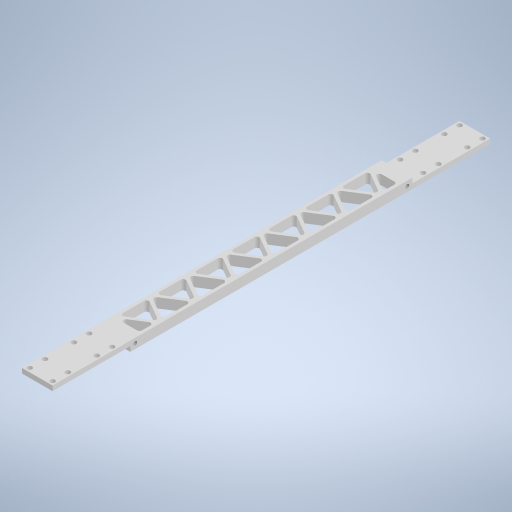
# Autodesk Inventor part: Connector Plate
Saved by Autodesk Inventor 2023 (Build 270158000, 158)
## iProperties
Created: 2022-09-25
Part Number: Connector Plate
Material: Generic
Document SubType Name: Modeling
Designer: deli
Density: 1 g/cm^3
Appearance: Default
Author: deli
Autodesk Inventor part; units mm, degrees
ref_plane "YZ Plane" through (0, 0, 0) normal (1, 0, 0) x (0, 1, 0)
ref_plane "XZ Plane" through (0, 0, 0) normal (0, 1, 0) x (-1, 0, 0)
ref_plane "XY Plane" through (0, 0, 0) normal (0, 0, 1) x (1, 0, 0)
sketch "Sketch1" plane through (0, 0, 0) normal (0, 1, 0) x (-1, 0, 0)
  line L0 (25.6456, 316.5178) -> (5.6456, 316.5178)
  line L1 (5.6456, 316.5178) -> (5.6456, 30.4178)
  line L2 (5.6456, 30.4178) -> (25.6456, 30.4178)
  line L3 (25.6456, 30.4178) -> (25.6456, 316.5178)
  circle A0 centre (23.1456, 314.0178) radius 1.6
  circle A1 centre (23.1456, 304.0178) radius 1.6
  circle A2 centre (8.1456, 314.0178) radius 1.6
  circle A3 centre (8.1456, 304.0178) radius 1.6
  line L4 (23.1456, 314.0178) -> (23.1456, 304.0178) construction
  line L5 (23.1456, 304.0178) -> (8.1456, 304.0178) construction
  line L6 (8.1456, 304.0178) -> (8.1456, 314.0178) construction
  line L7 (8.1456, 314.0178) -> (23.1456, 314.0178) construction
  circle A4 centre (23.1456, 285.1178) radius 1.6
  circle A5 centre (23.1456, 275.1178) radius 1.6
  circle A6 centre (8.1456, 285.1178) radius 1.6
  circle A7 centre (8.1456, 275.1178) radius 1.6
  line L8 (23.1456, 285.1178) -> (23.1456, 275.1178) construction
  line L9 (23.1456, 275.1178) -> (8.1456, 275.1178) construction
  line L10 (8.1456, 275.1178) -> (8.1456, 285.1178) construction
  line L11 (8.1456, 285.1178) -> (23.1456, 285.1178) construction
  circle A8 centre (23.1456, 71.8178) radius 1.6
  circle A9 centre (23.1456, 61.8178) radius 1.6
  circle A10 centre (8.1456, 71.8178) radius 1.6
  circle A11 centre (8.1456, 61.8178) radius 1.6
  line L12 (23.1456, 71.8178) -> (23.1456, 61.8178) construction
  line L13 (23.1456, 61.8178) -> (8.1456, 61.8178) construction
  line L14 (8.1456, 61.8178) -> (8.1456, 71.8178) construction
  line L15 (8.1456, 71.8178) -> (23.1456, 71.8178) construction
  circle A12 centre (23.1456, 42.9178) radius 1.6
  circle A13 centre (23.1456, 32.9178) radius 1.6
  circle A14 centre (8.1456, 42.9178) radius 1.6
  circle A15 centre (8.1456, 32.9178) radius 1.6
  line L16 (23.1456, 42.9178) -> (23.1456, 32.9178) construction
  line L17 (23.1456, 32.9178) -> (8.1456, 32.9178) construction
  line L18 (8.1456, 32.9178) -> (8.1456, 42.9178) construction
  line L19 (8.1456, 42.9178) -> (23.1456, 42.9178) construction
  line L20 (7.6456, 76.6425) -> (23.6456, 76.6425)
  line L21 (23.6456, 89.1783) -> (7.6456, 79.0121)
  line L22 (7.6456, 76.6425) -> (7.6456, 269.3043) construction
  line L23 (23.6456, 76.6425) -> (23.6456, 269.3043) construction
  line L24 (7.6456, 269.3043) -> (23.6456, 269.3043)
  line L25 (23.6456, 89.1783) -> (7.6456, 98.4159)
  line L26 (7.6456, 79.0121) -> (7.6456, 98.4159)
  line L27 (23.6456, 91.4877) -> (7.6456, 100.7253)
  line L28 (23.6456, 110.8914) -> (7.6456, 100.7253)
  line L29 (23.6456, 91.4877) -> (23.6456, 110.8914)
  line L30 (7.6456, 103.0948) -> (23.6456, 113.261)
  line L31 (23.6456, 113.261) -> (7.6456, 122.4986)
  line L32 (7.6456, 122.4986) -> (7.6456, 103.0948)
  line L33 (23.6456, 115.5704) -> (7.6456, 124.808)
  line L34 (7.6456, 124.808) -> (23.6456, 134.9741)
  line L35 (23.6456, 134.9741) -> (23.6456, 115.5704)
  line L36 (23.6456, 137.3437) -> (7.6456, 127.1775)
  line L37 (7.6456, 127.1775) -> (7.6456, 146.5813)
  line L38 (23.6456, 137.3437) -> (7.6456, 146.5813)
  line L39 (23.6456, 139.6531) -> (7.6456, 148.8907)
  line L40 (7.6456, 148.8907) -> (23.6456, 159.0568)
  line L41 (23.6456, 159.0568) -> (23.6456, 139.6531)
  line L42 (7.6456, 151.2603) -> (23.6456, 161.4264)
  line L43 (23.6456, 161.4264) -> (7.6456, 170.664)
  line L44 (7.6456, 151.2603) -> (7.6456, 170.664)
  line L45 (7.6456, 172.9734) -> (23.6456, 163.7358)
  line L46 (23.6456, 163.7358) -> (23.6456, 183.1396)
  line L47 (23.6456, 183.1396) -> (7.6456, 172.9734)
  line L48 (7.6456, 175.343) -> (23.6456, 185.5091)
  line L49 (23.6456, 185.5091) -> (7.6456, 194.7467)
  line L50 (7.6456, 175.343) -> (7.6456, 194.7467)
  line L51 (7.6456, 76.6425) -> (23.6456, 86.8087)
  line L52 (23.6456, 187.8185) -> (7.6456, 197.0561)
  line L53 (7.6456, 197.0561) -> (23.6456, 207.2223)
  line L54 (23.6456, 187.8185) -> (23.6456, 207.2223)
  line L55 (23.6456, 209.5918) -> (7.6456, 199.4257)
  line L56 (7.6456, 199.4257) -> (7.6456, 218.8294)
  line L57 (7.6456, 218.8294) -> (23.6456, 209.5918)
  line L58 (23.6456, 211.9012) -> (7.6456, 221.1388)
  line L59 (7.6456, 221.1388) -> (23.6456, 231.305)
  line L60 (23.6456, 231.305) -> (23.6456, 205.5717)
  line L61 (7.6456, 223.5084) -> (23.6456, 233.6746)
  line L62 (23.6456, 233.6746) -> (7.6456, 242.9122)
  line L63 (7.6456, 242.9122) -> (7.6456, 223.5084)
  line L64 (7.6456, 245.2216) -> (23.6456, 235.984)
  line L65 (23.6456, 235.984) -> (23.6456, 255.3877)
  line L66 (23.6456, 255.3877) -> (7.6456, 245.2216)
  line L67 (7.6456, 247.5911) -> (23.6456, 257.7573)
  line L68 (23.6456, 257.7573) -> (7.6456, 266.9949)
  line L69 (7.6456, 266.9949) -> (7.6456, 247.5911)
  line L70 (23.6456, 269.3043) -> (23.6456, 260.0667)
  line L71 (23.6456, 260.0667) -> (7.6456, 269.3043)
  line L72 (23.6456, 76.6425) -> (23.6456, 86.8087)
  line L73 (23.1456, 32.9178) -> (8.1456, 42.9178) construction
  line L74 (8.1456, 32.9178) -> (23.1456, 42.9178) construction
  line L75 (23.1456, 42.9178) -> (8.1456, 61.8178) construction
  line L76 (8.1456, 61.8178) -> (23.1456, 71.8178) construction
  line L77 (8.1456, 71.8178) -> (23.1456, 61.8178) construction
  line L78 (19.5805, 32.4178) -> (11.7107, 32.4178)
  line L79 (7.6456, 36.4829) -> (7.6456, 39.3527)
  line L80 (23.6456, 39.3527) -> (23.6456, 36.4829)
  arc A16 (7.6456, 68.2527) -> (7.6456, 75.3829) centre (8.1456, 71.8178) ccw
  arc A17 (23.6456, 75.3829) -> (23.6456, 68.2527) centre (23.1456, 71.8178) ccw
  line L81 (23.6456, 58.2527) -> (23.6456, 46.4829)
  line L82 (7.6456, 46.4829) -> (7.6456, 58.2527)
  line L83 (7.6456, 65.3829) -> (7.6456, 68.2527)
  line L84 (23.6456, 68.2527) -> (23.6456, 65.3829)
  arc A18 (23.6456, 307.5829) -> (23.6456, 300.4527) centre (23.1456, 304.0178) ccw
  arc A19 (7.6456, 310.4527) -> (11.7107, 314.5178) centre (8.1456, 314.0178) ccw
  arc A20 (7.6456, 300.4527) -> (7.6456, 307.5829) centre (8.1456, 304.0178) ccw
  arc A21 (23.6456, 288.6829) -> (23.6456, 281.5527) centre (23.1456, 285.1178) ccw
  arc A22 (23.6456, 278.6829) -> (23.6456, 271.5527) centre (23.1456, 275.1178) ccw
  arc A23 (7.6456, 271.5527) -> (7.6456, 278.6829) centre (8.1456, 275.1178) ccw
  arc A24 (7.6456, 281.5527) -> (7.6456, 288.6829) centre (8.1456, 285.1178) ccw
  line L85 (23.6456, 271.5527) -> (23.6456, 75.3829)
  line L86 (23.6456, 281.5527) -> (23.6456, 278.6829)
  line L87 (23.6456, 310.4527) -> (23.6456, 307.5829)
  line L88 (23.6456, 300.4527) -> (23.6456, 288.6829)
  arc A25 (19.5805, 314.5178) -> (23.6456, 310.4527) centre (23.1456, 314.0178) ccw
  line L89 (11.7107, 314.5178) -> (19.5805, 314.5178)
  line L90 (7.6456, 307.5829) -> (7.6456, 310.4527)
  line L91 (7.6456, 288.6829) -> (7.6456, 300.4527)
  line L92 (7.6456, 278.6829) -> (7.6456, 281.5527)
  line L93 (7.6456, 75.3829) -> (7.6456, 271.5527)
  arc A26 (23.6456, 36.4829) -> (20.8228, 35.6681) centre (23.1456, 32.9178) ccw
  arc A27 (19.7134, 34.004) -> (19.5805, 32.4178) centre (23.1456, 32.9178) ccw
  line L94 (20.8228, 40.1674) -> (17.4484, 37.9178)
  line L95 (15.6456, 36.7159) -> (11.5778, 34.004)
  line L96 (10.4684, 35.6681) -> (13.8428, 37.9178)
  line L97 (15.6456, 39.1196) -> (19.7134, 41.8315)
  line L98 (20.8228, 35.6681) -> (17.4484, 37.9178)
  line L99 (15.6456, 39.1196) -> (11.5778, 41.8315)
  line L100 (19.7134, 34.004) -> (15.6456, 36.7159)
  line L101 (13.8428, 37.9178) -> (10.4684, 40.1674)
  arc A28 (11.7107, 32.4178) -> (11.5778, 34.004) centre (8.1456, 32.9178) ccw
  arc A29 (10.4684, 35.6681) -> (7.6456, 36.4829) centre (8.1456, 32.9178) ccw
  arc A30 (7.6456, 39.3527) -> (10.4684, 40.1674) centre (8.1456, 42.9178) ccw
  arc A31 (20.8228, 40.1674) -> (23.6456, 39.3527) centre (23.1456, 42.9178) ccw
  line L102 (8.1456, 42.9178) -> (23.1456, 61.8178) construction
  line L103 (21.779, 46.2483) -> (16.9222, 52.3678)
  line L104 (15.6456, 53.9764) -> (11.0788, 59.7306)
  line L105 (11.0788, 45.005) -> (15.6456, 50.7592)
  line L106 (16.9222, 52.3678) -> (21.779, 58.4872)
  line L107 (20.2124, 45.005) -> (15.6456, 50.7592)
  line L108 (14.3689, 52.3678) -> (9.5122, 58.4872)
  line L109 (20.2124, 59.7306) -> (15.6456, 53.9764)
  line L110 (14.3689, 52.3678) -> (9.5122, 46.2483)
  arc A32 (23.6456, 46.4829) -> (21.779, 46.2483) centre (23.1456, 42.9178) ccw
  arc A33 (20.2124, 45.005) -> (19.7134, 41.8315) centre (23.1456, 42.9178) ccw
  arc A34 (11.5778, 41.8315) -> (11.0788, 45.005) centre (8.1456, 42.9178) ccw
  arc A35 (9.5122, 46.2483) -> (7.6456, 46.4829) centre (8.1456, 42.9178) ccw
  arc A36 (7.6456, 58.2527) -> (9.5122, 58.4872) centre (8.1456, 61.8178) ccw
  arc A37 (11.0788, 59.7306) -> (7.6456, 65.3829) centre (8.1456, 61.8178) ccw
  arc A38 (23.6456, 65.3829) -> (20.2124, 59.7306) centre (23.1456, 61.8178) ccw
  arc A39 (21.779, 58.4872) -> (23.6456, 58.2527) centre (23.1456, 61.8178) ccw
  line L111 (23.6456, 89.2678) -> (7.3765, 89.2678)
  line L112 (23.6456, 257.6678) -> (7.6456, 257.6678)
  point P0 (0, 0)
  point P1 (15.6456, 216.52)
  point P2 (15.6456, 264.6855)
  point P3 (23.6456, 211.9012)
  point P4 (15.6456, 30.4178)
  point P5 (7.6456, 257.6678)
  point P6 (16.8724, 261.6678)
  point P7 (17.491, 85.2678)
  point P8 (7.6456, 89.2678)
  point P9 (15.511, 89.2678)
  point P10 (23.5047, 257.6678)
  point P11 (23.4905, 89.2678)
  dimension "d0" = 20
  dimension "d23" = 3.2
  dimension "d24" = 3.2
  dimension "d25" = 3.2
  dimension "d26" = 3.2
  dimension "d27" = 15
  dimension "d28" = 10
  dimension "d29" = 2.5
  dimension "d31" = 3.2
  dimension "d32" = 3.2
  dimension "d33" = 3.2
  dimension "d34" = 3.2
  dimension "d35" = 10
  dimension "d36" = 15
  dimension "d37" = 2.5
  dimension "d38" = 18.9
  dimension "d45" = 3.2
  dimension "d46" = 3.2
  dimension "d47" = 3.2
  dimension "d48" = 3.2
  dimension "d49" = 10
  dimension "d50" = 15
  dimension "d54" = 3.2
  dimension "d55" = 3.2
  dimension "d56" = 3.2
  dimension "d57" = 3.2
  dimension "d58" = 10
  dimension "d59" = 15
  dimension "d63" = 18.9
  dimension "d64" = 2.5
  dimension "d65" = 2.5
  dimension "d68" = 2
  dimension "d73" = 60
  dimension "d74" = 2
  dimension "d75" = 2
  dimension "d76" = 2
  dimension "d77" = 2
  dimension "d78" = 2
  dimension "d79" = 2
  dimension "d80" = 2
  dimension "d81" = 2
  dimension "d82" = 2
  dimension "d83" = 192.6617
  dimension "d84" = 2
  dimension "d86" = 2
  dimension "d87" = 2
  dimension "d88" = 2
  dimension "d89" = 2
  dimension "d90" = 2
  dimension "d92" = 2.3094
  dimension "d93" = 2
  dimension "d94" = 203.3
  dimension "d96" = 2
  dimension "d101" = 281.1
  dimension "d107" = 2.5
  dimension "d108" = 2.5
  dimension "d111" = 2
  dimension "d112" = 2
  dimension "d114" = 2
  dimension "d118" = 2
  dimension "d119" = 2
  dimension "d121" = 2
  dimension "d122" = 2
  dimension "d124" = 2
  constraints: 222 end point, 99 parallel, 48 point on circle, 40 centre point, 20 perpendicular, 16 coincident, 15 vertical, 6 horizontal, 4 midpoint, 4 point on line, 1 concentric, 54 other
  measures "d0" distance of L2.end L1.end
  measures "d23" diameter of A0
  measures "d24" diameter of A1
  measures "d25" diameter of A2
  measures "d26" diameter of A3
  measures "d27" distance of L6.end L4.start
  measures "d28" distance of L4.start L4.end
  measures "d29" distance from line of L1 L6.end
  measures "d31" diameter of A4
  measures "d32" diameter of A5
  measures "d33" diameter of A6
  measures "d34" diameter of A7
  measures "d35" distance of L8.start L8.end
  measures "d36" distance of L10.end L8.start
  measures "d37" distance from line of L1 L10.end
  measures "d38" distance of L10.end L5.end
  measures "d45" diameter of A8
  measures "d46" diameter of A9
  measures "d47" diameter of A10
  measures "d48" diameter of A11
  measures "d49" distance of L15.end L12.end
  measures "d50" distance of L15.start L15.end
  measures "d54" diameter of A12
  measures "d55" diameter of A13
  measures "d56" diameter of A14
  measures "d57" diameter of A15
  measures "d58" distance of L19.end L16.end
  measures "d59" distance of L19.start L19.end
  measures "d63" distance of L14.start L19.start
  measures "d64" distance from line of L1 L15.start
  measures "d65" distance from line of L1 L19.start
  measures "d68" distance from line of L20.start L1
  measures "d73" angle of L25 L26
  measures "d74" distance between parallel lines of L27 L25
  measures "d75" distance between parallel lines of L30 L28
  measures "d76" distance between parallel lines of L33 L31
  measures "d77" distance between parallel lines of L36 L34
  measures "d78" distance between parallel lines of L39 L38
  measures "d79" distance between parallel lines of L40 L42
  measures "d80" distance between parallel lines of L43 L45
  measures "d81" distance between parallel lines of L48 L47
  measures "d82" distance between parallel lines of L21 L51
  measures "d83" distance between parallel lines of L24 L20
  measures "d84" distance between parallel lines of L52 L49
  measures "d86" distance between parallel lines of L55 L53
  measures "d87" distance from line of point (15.646, 216.52) L57
  measures "d88" distance between parallel lines of L59 L61
  measures "d89" distance between parallel lines of L64 L62
  measures "d90" distance between parallel lines of L66 L67
  measures "d92" distance from line of L24 L68.end
  measures "d93" distance from line of point (15.646, 264.685) L68
  measures "d94" distance between parallel lines of L15 L9
  measures "d101" distance of L18.start L6.end
  measures "d107" distance from line of point (15.646, 30.418) L17
  measures "d108" distance between parallel lines of L0 L7
  measures "d111" distance between parallel lines of L2 L78
  measures "d112" distance between parallel lines of L3 L80
  measures "d114" distance between parallel lines of L1 L79
  measures "d118" radial gap between concentric circles of A17 A8
  measures "d119" radial gap between concentric circles of A10 A16
  measures "d121" distance between parallel lines of L3 L81
  measures "d122" distance between parallel lines of L3 L84
  measures "d124" distance between parallel lines of L1 L82
extrude "Extrusion1" add sketch "Sketch1" along normal blind 6.35 contours L3 L2 L1 L0 | L51 L72 L20 | L93 L21 L85 L51 | L20 L85 A17 L84 A38 L109 L104 A37 L83 A16 L93 | L26 L111 L25 L21 | L25 L111 L85 | L25 L93 L27 L85 L111 | L93 L30 L85 L28 | L31 L93 L33 L85 | L93 L36 L85 L34 | L38 L93 L39 L85 | L93 L42 L85 L40 | L43 L93 L45 L85 | L93 L48 L85 L47 | L49 L93 L52 L85 | L93 L55 L60 L53 | L57 L93 L58 L60 | L93 L61 L85 L59 | L62 L93 L64 L85 | L93 L67 L112 L85 L66 | L112 L67 L85 | L112 L69 L68 L67 | L68 L93 L71 L85 | L71 L24 L70 | L93 A23 L92 A24 L91 A20 L90 A19 L89 A25 L87 A18 L88 A21 L86 A22 L85 L24 | L78 A28 L95 L100 A27 | L79 A30 L101 L96 A29 | L80 A26 L98 L94 A31 | L81 A32 L103 L106 A39 | L82 A36 L108 L110 A35 | L99 A34 L105 L107 A33 L97
fillet "Fillet1" radius 1.5875 45 edges at (-7.6456, 3.175, 247.5911) (-7.6456, 3.175, 245.2216) (-7.6456, 3.175, 242.9122) (-23.6456, 3.175, 255.3877) (-23.6456, 3.175, 235.984) (-23.6456, 3.175, 233.6746) (-7.6456, 3.175, 223.5084) (-23.6456, 3.175, 231.305) (-7.6456, 3.175, 221.1388) (-23.6456, 3.175, 211.9012) (-23.6456, 3.175, 209.5918) (-7.6456, 3.175, 218.8294) (-7.6456, 3.175, 199.4257) (-23.6456, 3.175, 207.2223) (-7.6456, 3.175, 197.0561) (-23.6456, 3.175, 187.8185) (-23.6456, 3.175, 185.5091) (-7.6456, 3.175, 194.7467) (-7.6456, 3.175, 175.343) (-23.6456, 3.175, 183.1396) (-7.6456, 3.175, 172.9734) (-23.6456, 3.175, 163.7358) (-23.6456, 3.175, 161.4264) (-7.6456, 3.175, 170.664) (-7.6456, 3.175, 151.2603) (-23.6456, 3.175, 159.0568) (-7.6456, 3.175, 148.8907) (-23.6456, 3.175, 139.6531) (-23.6456, 3.175, 137.3437) (-7.6456, 3.175, 146.5813) (-7.6456, 3.175, 127.1775) (-7.6456, 3.175, 124.808) (-23.6456, 3.175, 134.9741) (-23.6456, 3.175, 115.5704) (-23.6456, 3.175, 113.261) (-7.6456, 3.175, 122.4986) (-7.6456, 3.175, 103.0948) (-7.6456, 3.175, 100.7253) (-23.6456, 3.175, 110.8914) (-23.6456, 3.175, 91.4877) (-7.6456, 3.175, 98.4159) (-7.6456, 3.175, 89.2678) (-7.6456, 3.175, 257.6678) (-23.4905, 3.175, 89.2678) (-23.5047, 3.175, 257.6678)
sketch "Sketch2" plane through (0, 6.35, 0) normal (0, 1, 0) x (1, 0, 0)
  line L0 (-5.6456, -30.4178) -> (-25.6456, -30.4178) projected
  line L1 (-5.6456, -316.5178) -> (-5.6456, -30.4178) projected
  line L2 (-25.6456, -30.4178) -> (-5.6456, -30.4178)
  line L3 (-5.6456, -30.4178) -> (-5.6456, -81.2678)
  line L4 (-5.6456, -81.2678) -> (-25.6456, -81.2678)
  line L5 (-25.6456, -81.2678) -> (-25.6456, -30.4178)
  point P0 (0, 0)
  dimension "d182" = 50.85
  constraints: 8 end point, 2 parallel, 1 horizontal, 1 perpendicular, 1 point on line
  measures "d182" distance of L2.end L3.end
extrude "Extrusion2" cut sketch "Sketch2" against normal blind 3.175
sketch "Sketch3" plane through (0, 0, 0) normal (0, -1, 0) x (1, 0, 0)
  line L0 (-25.6456, 30.4178) -> (-25.6456, 316.5178) projected
  line L1 (-5.6456, 316.5178) -> (-5.6456, 30.4178) projected
  line L2 (-25.6456, 316.5178) -> (-5.6456, 316.5178)
  line L3 (-5.6456, 316.5178) -> (-5.6456, 265.6678)
  line L4 (-5.6456, 265.6678) -> (-25.6456, 265.6678)
  line L5 (-25.6456, 265.6678) -> (-25.6456, 316.5178)
  point P0 (0, 0)
  point P1 (-5.6456, 316.5178)
  point P2 (-25.6456, 265.6678)
  dimension "d192" = 50.85
  constraints: 8 end point, 2 parallel, 1 horizontal, 1 perpendicular, 1 point on line
  measures "d192" distance of L2.end L3.end
extrude "Extrusion3" cut sketch "Sketch3" against normal blind 3.175
sketch "Sketch4" plane through (-5.6456, 6.35, 316.5178) normal (1, 0, 0) x (0, 0, -1)
  circle A0 centre (232, -3.175) radius 1.25
  line L0 (50.85, -6.35) -> (286.1, -6.35) projected
  line L1 (235.25, -3.175) -> (235.25, 0) projected
  circle A1 centre (54.1, -3.175) radius 1.25
  line L2 (50.85, -3.175) -> (50.85, -6.35) projected
  point P0 (316.5178, -6.35)
  dimension "d196" = 2.5
  dimension "d199" = 2
  dimension "d200" = 3.175
  dimension "d207" = 2.5
  dimension "d208" = 2
  dimension "d209" = 3.175
  constraints: 2 centre point
  measures "d196" diameter of A0
  measures "d199" distance edge to line of A0 L1
  measures "d200" distance from line of L0 A0.centre
  measures "d207" diameter of A1
  measures "d208" distance edge to line of A1 L2
  measures "d209" distance from line of A1.centre L0
extrude "Extrusion4" cut sketch "Sketch4" against normal blind 8
thread "Thread1" size "M3x0.5" class "6H" standard "ANSI Metric M Profile" full length
thread "Thread3" size "M3x0.5" class "6H" standard "ANSI Metric M Profile" full length
equation "\"d24\" = d23"
equation "\"d25\" = d23"
equation "\"d26\" = d23"
equation "\"d29\" = -0.5 * d27 + 0.5 * d0"
equation "\"d31\" = d23"
equation "\"d32\" = d23"
equation "\"d33\" = d23"
equation "\"d34\" = d23"
equation "\"d35\" = d28"
equation "\"d36\" = d27"
equation "\"d37\" = d29"
equation "\"d45\" = d51"
equation "\"d46\" = d51"
equation "\"d47\" = d51"
equation "\"d48\" = d51"
equation "\"d49\" = d52"
equation "\"d50\" = d53"
equation "\"d54\" = d60"
equation "\"d55\" = d60"
equation "\"d56\" = d60"
equation "\"d57\" = d60"
equation "\"d58\" = d61"
equation "\"d59\" = d62"
equation "\"d63\" = d38"
equation "\"d64\" = d29"
equation "\"d65\" = d29"
equation "\"d74\" = d82"
equation "\"d75\" = d74"
equation "\"d76\" = d75"
equation "\"d77\" = d76"
equation "\"d78\" = d77"
equation "\"d79\" = d78"
equation "\"d80\" = d79"
equation "\"d81\" = d80"
equation "\"d84\" = d81"
equation "\"d86\" = d84"
equation "\"d87\" = d86"
equation "\"d51\" = 3.2"
equation "\"d52\" = 10"
equation "\"d53\" = 15"
equation "\"d60\" = 3.2"
equation "\"d61\" = 10"
equation "\"d62\" = 15"
body "Solid1"
